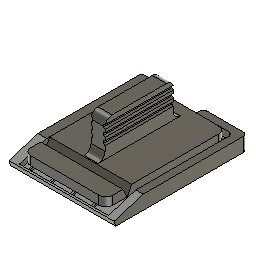
shadowmask_quadrant_cleaver (Autodesk Fusion 360 design; units mm, degrees)
Autodesk Fusion 360 part; units mm, degrees
note: some values were not read from the file. Chosen so that the rebuilt part matches the saved one: a direction; which face or edge a step refers to. Set by a fixed rule: which sketch regions a step uses.
sketch "Sketch1" plane through (0, 0, 0) normal (0, 0, 1) x (1, 0, 0)
  line L0 (39.6677, 30.4381) -> (40.9576, 28.6788)
  line L1 (46.9846, 17.101) -> (47.6858, 15.0353)
  line L2 (10.822, 48.8148) -> (12.941, 48.2963)
  line L3 (35.3553, 35.3553) -> (36.8639, 33.7795)
  line L4 (30.5, 19) -> (26.5, 19)
  line L5 (5.5, 7) -> (5.5, 13)
  line L6 (28.6788, 40.9576) -> (30.4381, 39.6677)
  line L7 (33.7795, 36.8639) -> (35.3553, 35.3553)
  line L8 (4.3578, 49.8097) -> (6.5263, 49.5722)
  line L9 (50, 0) -> (0, 0)
  line L10 (32.1394, 38.3022) -> (33.7795, 36.8639)
  line L11 (2.181, 49.9524) -> (4.3578, 49.8097)
  line L12 (19.1342, 46.194) -> (21.1309, 45.3154)
  line L13 (48.8148, 10.822) -> (49.2404, 8.6824)
  line L14 (12.941, 48.2963) -> (15.0353, 47.6858)
  line L15 (48.2963, 12.941) -> (48.8148, 10.822)
  line L16 (5.5, 13) -> (9.5, 13)
  line L17 (17.101, 46.9846) -> (19.1342, 46.194)
  line L18 (44.3505, 23.0874) -> (45.3154, 21.1309)
  line L19 (49.2404, 8.6824) -> (49.5722, 6.5263)
  line L20 (6.5263, 49.5722) -> (8.6824, 49.2404)
  line L21 (30.4381, 39.6677) -> (32.1394, 38.3022)
  line L22 (0, 0) -> (0, 50)
  line L23 (43.3013, 25) -> (44.3505, 23.0874)
  line L24 (26.5, 19) -> (26.5, 25)
  line L25 (23.0874, 44.3505) -> (25, 43.3013)
  line L26 (42.1696, 26.865) -> (43.3013, 25)
  line L27 (38.3022, 32.1394) -> (39.6677, 30.4381)
  line L28 (49.9524, 2.181) -> (50, 0)
  line L29 (26.5, 25) -> (30.5, 25)
  line L30 (30.5, 25) -> (30.5, 19)
  line L31 (36.8639, 33.7795) -> (38.3022, 32.1394)
  line L32 (21.1309, 45.3154) -> (23.0874, 44.3505)
  line L33 (0, 50) -> (2.181, 49.9524)
  line L34 (46.194, 19.1342) -> (46.9846, 17.101)
  line L35 (40.9576, 28.6788) -> (42.1696, 26.865)
  line L36 (8.6824, 49.2404) -> (10.822, 48.8148)
  line L37 (9.5, 7) -> (5.5, 7)
  line L38 (49.5722, 6.5263) -> (49.8097, 4.3578)
  line L39 (49.8097, 4.3578) -> (49.9524, 2.181)
  line L40 (26.865, 42.1696) -> (28.6788, 40.9576)
  line L41 (47.6858, 15.0353) -> (48.2963, 12.941)
  line L42 (25, 43.3013) -> (26.865, 42.1696)
  line L43 (45.3154, 21.1309) -> (46.194, 19.1342)
  line L44 (15.0353, 47.6858) -> (17.101, 46.9846)
  line L45 (9.5, 13) -> (9.5, 7)
  line L46 (25.0885, 2) -> (24.9115, 2)
  line L47 (17.9115, 4.0885) -> (18.0885, 4.0885)
  line L48 (45.9115, 3.9115) -> (39.0885, 3.9115)
  line L49 (38.9115, 15.9115) -> (32.0885, 15.9115)
  line L50 (45.2548, 15.9115) -> (39.0885, 15.9115)
  line L51 (3.9115, 27.9115) -> (2, 27.9115)
  line L52 (2, 39.9115) -> (3.9115, 39.9115)
  line L53 (10.9115, 16.0885) -> (11.0885, 16.0885)
  line L54 (38.9872, 27.9821) -> (39.0885, 27.9821)
  line L55 (3.9115, 16.0885) -> (3.9115, 27.9115)
  line L56 (2, 4.0885) -> (3.9115, 4.0885)
  line L57 (25.0885, 28.0885) -> (31.9115, 28.0885)
  line L58 (4.0885, 39.9115) -> (10.9115, 39.9115)
  line L59 (26.533, 40.0885) -> (26.533, 39.9115)
  line L60 (24.9115, 16.0885) -> (24.9115, 15.9115)
  line L61 (25.0885, 39.9115) -> (25.0885, 28.0885)
  line L62 (11.0885, 28.0885) -> (17.9115, 28.0885)
  line L63 (45.9115, 2) -> (45.9115, 3.9115)
  line L64 (11.0885, 27.9115) -> (17.9115, 27.9115)
  line L65 (10.9115, 28.0885) -> (10.9115, 39.9115)
  line L66 (17.9115, 39.9115) -> (11.0885, 39.9115)
  line L67 (4.0885, 39.9115) -> (4.0885, 28.0885)
  line L68 (10.9115, 15.9115) -> (11.0885, 15.9115)
  line L69 (31.9115, 16.0885) -> (31.9115, 27.9115)
  line L70 (18.0885, 39.9115) -> (18.0885, 28.0885)
  line L71 (3.9115, 28.0885) -> (3.9115, 39.9115)
  line L72 (3.9115, 16.0885) -> (3.9115, 15.9115)
  line L73 (32.0885, 4.0885) -> (38.9115, 4.0885)
  line L74 (10.9115, 16.0885) -> (10.9115, 27.9115)
  line L75 (2, 3.9115) -> (2, 4.0885)
  line L76 (4.0885, 15.9115) -> (4.0885, 4.0885)
  line L77 (4.0885, 16.0885) -> (3.9115, 16.0885)
  line L78 (38.9872, 27.9115) -> (38.9872, 27.9821)
  line L79 (39.0885, 4.0885) -> (38.9115, 4.0885)
  line L80 (3.9115, 47.833) -> (4.0885, 47.833)
  line L81 (10.9115, 4.0885) -> (11.0885, 4.0885)
  line L82 (4.0885, 28.0885) -> (10.9115, 28.0885)
  line L83 (4.0885, 27.9115) -> (10.9115, 27.9115)
  line L84 (3.9115, 4.0885) -> (4.0885, 4.0885)
  line L85 (18.0885, 40.0885) -> (17.9115, 40.0885)
  line L86 (2, 39.9115) -> (2, 40.0885)
  line L87 (4.0885, 4.0885) -> (10.9115, 4.0885)
  line L88 (11.0885, 39.9115) -> (17.9115, 39.9115)
  line L89 (38.9115, 3.9115) -> (32.0885, 3.9115)
  line L90 (39.0885, 16.0885) -> (38.9115, 16.0885)
  line L91 (17.9115, 16.0885) -> (17.9115, 27.9115)
  line L92 (10.9115, 15.9115) -> (4.0885, 15.9115)
  line L93 (4.0885, 40.0885) -> (10.9115, 40.0885)
  line L94 (31.9115, 15.9115) -> (25.0885, 15.9115)
  line L95 (18.0885, 15.9115) -> (18.0885, 4.0885)
  line L96 (25.0885, 27.9115) -> (25.0885, 16.0885)
  line L97 (11.0885, 4.0885) -> (10.9115, 4.0885)
  line L98 (11.0885, 15.9115) -> (11.0885, 4.0885)
  line L99 (39.0885, 3.9115) -> (39.0885, 4.0885)
  line L100 (4.0885, 15.9115) -> (4.0885, 16.0885)
  line L101 (11.0885, 40.0885) -> (17.9115, 40.0885)
  line L102 (24.9115, 3.9115) -> (18.0885, 3.9115)
  line L103 (11.0885, 40.0885) -> (10.9115, 40.0885)
  line L104 (18.0885, 4.0885) -> (17.9115, 4.0885)
  line L105 (18.0885, 16.0885) -> (24.9115, 16.0885)
  line L106 (24.9115, 39.9115) -> (25.0885, 39.9115)
  line L107 (10.9115, 40.0885) -> (10.9115, 46.7226)
  line L108 (32.0885, 2) -> (31.9115, 2)
  line L109 (31.9115, 4.0885) -> (32.0885, 4.0885)
  line L110 (10.9115, 27.9115) -> (4.0885, 27.9115)
  line L111 (24.9115, 3.9115) -> (18.0885, 3.9115)
  line L112 (18.0885, 15.9115) -> (18.0885, 16.0885)
  line L113 (11.0885, 16.0885) -> (10.9115, 16.0885)
  line L114 (38.9115, 27.9115) -> (32.0885, 27.9115)
  line L115 (31.9115, 16.0885) -> (31.9115, 15.9115)
  line L116 (10.9115, 39.9115) -> (4.0885, 39.9115)
  line L117 (25.0885, 27.9115) -> (25.0885, 28.0885)
  line L118 (31.9115, 28.0885) -> (31.9115, 27.9115)
  line L119 (39.0885, 4.0885) -> (45.9115, 4.0885)
  line L120 (32.0885, 15.9115) -> (32.0885, 16.0885)
  line L121 (3.9115, 4.0885) -> (3.9115, 3.9115)
  line L122 (3.9115, 16.0885) -> (4.0885, 16.0885)
  line L123 (25.0885, 39.9115) -> (25.0885, 40.0885)
  line L124 (18.0885, 28.0885) -> (24.9115, 28.0885)
  line L125 (17.9115, 28.0885) -> (17.9115, 27.9115)
  line L126 (24.9115, 27.9115) -> (18.0885, 27.9115)
  line L127 (38.9115, 27.9821) -> (38.9115, 27.9115)
  line L128 (17.9115, 28.0885) -> (17.9115, 39.9115)
  line L129 (18.0885, 16.0885) -> (17.9115, 16.0885)
  line L130 (32.0885, 28.0885) -> (31.9115, 28.0885)
  line L131 (18.0885, 16.0885) -> (17.9115, 16.0885)
  line L132 (10.9115, 28.0885) -> (10.9115, 27.9115)
  line L133 (38.9115, 16.0885) -> (38.9115, 27.9115)
  line L134 (17.9115, 44.4972) -> (18.0885, 44.4972)
  line L135 (24.9115, 28.0885) -> (24.9115, 27.9115)
  line L136 (24.9115, 15.9115) -> (18.0885, 15.9115)
  line L137 (38.9872, 28.0885) -> (38.9872, 27.9821)
  line L138 (18.0885, 39.9115) -> (18.0885, 40.0885)
  line L139 (39.0885, 15.9115) -> (39.0885, 4.0885)
  line L140 (10.9115, 16.0885) -> (10.9115, 15.9115)
  line L141 (24.9115, 40.9756) -> (25.0885, 40.9756)
  line L142 (4.0885, 4.0885) -> (3.9115, 4.0885)
  line L143 (18.0885, 27.9115) -> (18.0885, 16.0885)
  line L144 (4.0885, 40.0885) -> (3.9115, 40.0885)
  line L145 (32.0885, 4.0885) -> (31.9115, 4.0885)
  line L146 (17.9115, 40.0885) -> (17.9115, 44.4972)
  line L147 (31.9115, 27.9115) -> (25.0885, 27.9115)
  line L148 (25.0885, 27.9115) -> (31.9115, 27.9115)
  line L149 (38.9115, 3.9115) -> (32.0885, 3.9115)
  line L150 (2, 40.0885) -> (3.9115, 40.0885)
  line L151 (18.0885, 4.0885) -> (24.9115, 4.0885)
  line L152 (45.9115, 4.0885) -> (45.9115, 3.9115)
  line L153 (11.0885, 4.0885) -> (17.9115, 4.0885)
  line L154 (17.9115, 16.0885) -> (18.0885, 16.0885)
  line L155 (4.0885, 47.833) -> (4.0885, 40.0885)
  line L156 (4.0885, 3.9115) -> (4.0885, 4.0885)
  line L157 (4.0885, 28.0885) -> (3.9115, 28.0885)
  line L158 (17.9115, 27.9115) -> (11.0885, 27.9115)
  line L159 (10.9115, 39.9115) -> (11.0885, 39.9115)
  line L160 (47.833, 4.0885) -> (47.833, 3.9115)
  line L161 (24.9115, 16.0885) -> (24.9115, 27.9115)
  line L162 (11.0885, 16.0885) -> (10.9115, 16.0885)
  line L163 (17.9115, 15.9115) -> (18.0885, 15.9115)
  line L164 (17.9115, 4.0885) -> (17.9115, 3.9115)
  line L165 (38.9115, 27.9115) -> (32.0885, 27.9115)
  line L166 (18.0885, 3.9115) -> (18.0885, 4.0885)
  line L167 (31.9115, 3.9115) -> (25.0885, 3.9115)
  line L168 (4.0885, 16.0885) -> (10.9115, 16.0885)
  line L169 (3.9115, 15.9115) -> (4.0885, 15.9115)
  line L170 (3.9115, 39.9115) -> (4.0885, 39.9115)
  line L171 (10.9115, 15.9115) -> (4.0885, 15.9115)
  line L172 (25.0885, 15.9115) -> (25.0885, 16.0885)
  line L173 (10.9115, 3.9115) -> (4.0885, 3.9115)
  line L174 (24.9115, 16.0885) -> (25.0885, 16.0885)
  line L175 (18.0885, 28.0885) -> (17.9115, 28.0885)
  line L176 (4.0885, 15.9115) -> (10.9115, 15.9115)
  line L177 (10.9115, 27.9115) -> (11.0885, 27.9115)
  line L178 (25.0885, 40.0885) -> (26.533, 40.0885)
  line L179 (11.0885, 39.9115) -> (11.0885, 40.0885)
  line L180 (47.833, 3.9115) -> (46.0885, 3.9115)
  line L181 (25.0885, 3.9115) -> (25.0885, 4.0885)
  line L182 (11.0885, 46.7226) -> (11.0885, 40.0885)
  line L183 (38.9115, 15.9115) -> (39.0885, 15.9115)
  line L184 (24.9115, 4.0885) -> (24.9115, 3.9115)
  line L185 (25.0885, 16.0885) -> (31.9115, 16.0885)
  line L186 (31.9115, 3.9115) -> (25.0885, 3.9115)
  line L187 (25.0885, 16.0885) -> (24.9115, 16.0885)
  line L188 (10.9115, 4.0885) -> (10.9115, 3.9115)
  line L189 (46.0885, 4.0885) -> (47.833, 4.0885)
  line L190 (4.0885, 16.0885) -> (3.9115, 16.0885)
  line L191 (17.9115, 39.9115) -> (18.0885, 39.9115)
  line L192 (2, 27.9115) -> (3.9115, 27.9115)
  line L193 (11.0885, 28.0885) -> (10.9115, 28.0885)
  line L194 (32.0885, 27.9115) -> (38.9115, 27.9115)
  line L195 (24.9115, 15.9115) -> (25.0885, 15.9115)
  line L196 (2, 28.0885) -> (3.9115, 28.0885)
  line L197 (24.9115, 4.0885) -> (25.0885, 4.0885)
  line L198 (18.0885, 27.9115) -> (18.0885, 28.0885)
  line L199 (32.0885, 16.0885) -> (38.9115, 16.0885)
  line L200 (3.9115, 27.9115) -> (2, 27.9115)
  line L201 (32.0885, 35.7771) -> (32.0885, 28.0885)
  line L202 (38.9115, 16.0885) -> (38.9115, 15.9115)
  line L203 (25.0885, 28.0885) -> (24.9115, 28.0885)
  line L204 (25.0885, 4.0885) -> (24.9115, 4.0885)
  line L205 (2, 16.0885) -> (3.9115, 16.0885)
  line L206 (39.0885, 3.9115) -> (39.0885, 2)
  line L207 (10.9115, 39.9115) -> (4.0885, 39.9115)
  line L208 (25.0885, 4.0885) -> (24.9115, 4.0885)
  line L209 (46.0885, 3.9115) -> (46.0885, 2)
  line L210 (3.9115, 28.0885) -> (3.9115, 27.9115)
  line L211 (24.9115, 4.0885) -> (24.9115, 15.9115)
  line L212 (10.9115, 27.9115) -> (4.0885, 27.9115)
  line L213 (17.9115, 15.9115) -> (11.0885, 15.9115)
  line L214 (32.0885, 27.9115) -> (32.0885, 28.0885)
  line L215 (4.0885, 28.0885) -> (3.9115, 28.0885)
  line L216 (17.9115, 15.9115) -> (11.0885, 15.9115)
  line L217 (10.9115, 46.7226) -> (11.0885, 46.7226)
  line L218 (38.9115, 2) -> (38.9115, 3.9115)
  line L219 (24.9115, 15.9115) -> (18.0885, 15.9115)
  line L220 (38.9115, 27.9115) -> (38.9872, 27.9115)
  line L221 (17.9115, 40.0885) -> (17.9115, 39.9115)
  line L222 (32.0885, 15.9115) -> (32.0885, 4.0885)
  line L223 (11.0885, 39.9115) -> (11.0885, 28.0885)
  line L224 (10.9115, 40.0885) -> (10.9115, 39.9115)
  line L225 (3.9115, 40.0885) -> (3.9115, 47.833)
  line L226 (31.9115, 27.9115) -> (25.0885, 27.9115)
  line L227 (31.9115, 16.0885) -> (32.0885, 16.0885)
  line L228 (38.9115, 3.9115) -> (39.0885, 3.9115)
  line L229 (24.9115, 28.0885) -> (24.9115, 39.9115)
  line L230 (3.9115, 4.0885) -> (3.9115, 15.9115)
  line L231 (24.9115, 27.9115) -> (25.0885, 27.9115)
  line L232 (24.9115, 40.0885) -> (24.9115, 39.9115)
  line L233 (4.0885, 27.9115) -> (4.0885, 16.0885)
  line L234 (46.0885, 4.0885) -> (45.9115, 4.0885)
  line L235 (18.0885, 28.0885) -> (17.9115, 28.0885)
  line L236 (17.9115, 27.9115) -> (11.0885, 27.9115)
  line L237 (24.9115, 2) -> (24.9115, 3.9115)
  line L238 (11.0885, 16.0885) -> (17.9115, 16.0885)
  line L239 (45.9115, 4.0885) -> (45.9115, 13.7113)
  line L240 (32.0885, 4.0885) -> (31.9115, 4.0885)
  line L241 (17.9115, 16.0885) -> (17.9115, 15.9115)
  line L242 (32.0885, 3.9115) -> (32.0885, 2)
  line L243 (32.0885, 16.0885) -> (31.9115, 16.0885)
  line L244 (3.9115, 27.9115) -> (4.0885, 27.9115)
  line L245 (11.0885, 15.9115) -> (17.9115, 15.9115)
  line L246 (39.0885, 2) -> (38.9115, 2)
  line L247 (17.9115, 28.0885) -> (18.0885, 28.0885)
  line L248 (2, 15.9115) -> (3.9115, 15.9115)
  line L249 (2, 15.9115) -> (2, 16.0885)
  line L250 (18.0885, 27.9115) -> (24.9115, 27.9115)
  line L251 (18.0885, 15.9115) -> (24.9115, 15.9115)
  line L252 (2, 27.9115) -> (2, 28.0885)
  line L253 (46.0885, 2) -> (45.9115, 2)
  line L254 (46.0885, 13.7113) -> (46.0885, 4.0885)
  line L255 (25.0885, 40.9756) -> (25.0885, 40.0885)
  line L256 (45.9115, 13.7113) -> (46.0885, 13.7113)
  line L257 (18.0885, 4.0885) -> (17.9115, 4.0885)
  line L258 (17.9115, 4.0885) -> (17.9115, 15.9115)
  line L259 (3.9115, 28.0885) -> (4.0885, 28.0885)
  line L260 (4.0885, 4.0885) -> (3.9115, 4.0885)
  line L261 (25.0885, 3.9115) -> (25.0885, 2)
  line L262 (17.9115, 27.9115) -> (18.0885, 27.9115)
  line L263 (24.9115, 39.9115) -> (18.0885, 39.9115)
  line L264 (18.0885, 44.4972) -> (18.0885, 40.0885)
  line L265 (32.0885, 3.9115) -> (32.0885, 4.0885)
  line L266 (38.9115, 4.0885) -> (38.9115, 3.9115)
  line L267 (17.9115, 3.9115) -> (11.0885, 3.9115)
  line L268 (31.9115, 27.9115) -> (32.0885, 27.9115)
  line L269 (3.9115, 15.9115) -> (2, 15.9115)
  line L270 (26.533, 39.9115) -> (25.0885, 39.9115)
  line L271 (11.0885, 3.9115) -> (11.0885, 4.0885)
  line L272 (32.0885, 28.0885) -> (38.9872, 28.0885)
  line L273 (31.9115, 28.0885) -> (31.9115, 35.7771)
  line L274 (3.9115, 15.9115) -> (2, 15.9115)
  line L275 (3.9115, 39.9115) -> (2, 39.9115)
  line L276 (4.0885, 39.9115) -> (4.0885, 40.0885)
  line L277 (24.9115, 27.9115) -> (18.0885, 27.9115)
  line L278 (25.0885, 15.9115) -> (25.0885, 4.0885)
  line L279 (4.0885, 27.9115) -> (4.0885, 28.0885)
  line L280 (11.0885, 15.9115) -> (11.0885, 16.0885)
  line L281 (39.0885, 27.9821) -> (39.0885, 16.0885)
  line L282 (31.9115, 4.0885) -> (31.9115, 15.9115)
  line L283 (31.9115, 15.9115) -> (32.0885, 15.9115)
  line L284 (24.9115, 40.0885) -> (24.9115, 40.9756)
  line L285 (25.0885, 4.0885) -> (31.9115, 4.0885)
  line L286 (11.0885, 4.0885) -> (10.9115, 4.0885)
  line L287 (45.9115, 3.9115) -> (46.0885, 3.9115)
  line L288 (31.9115, 15.9115) -> (25.0885, 15.9115)
  line L289 (11.0885, 27.9115) -> (11.0885, 16.0885)
  line L290 (39.0885, 15.9115) -> (39.0885, 16.0885)
  line L291 (3.9115, 3.9115) -> (2, 3.9115)
  line L292 (46.0885, 3.9115) -> (46.0885, 4.0885)
  line L293 (38.9872, 27.9821) -> (38.9115, 27.9821)
  line L294 (11.0885, 27.9115) -> (11.0885, 28.0885)
  line L295 (25.0885, 40.0885) -> (24.9115, 40.0885)
  line L296 (31.9115, 4.0885) -> (31.9115, 3.9115)
  line L297 (18.0885, 40.0885) -> (24.9115, 40.0885)
  line L298 (25.0885, 16.0885) -> (24.9115, 16.0885)
  line L299 (3.9115, 39.9115) -> (2, 39.9115)
  line L300 (32.0885, 16.0885) -> (31.9115, 16.0885)
  line L301 (31.9115, 35.7771) -> (32.0885, 35.7771)
  line L302 (39.0885, 16.0885) -> (45.2548, 16.0885)
  line L303 (25.0885, 15.9115) -> (31.9115, 15.9115)
  line L304 (45.2548, 16.0885) -> (45.2548, 15.9115)
  line L305 (11.0885, 28.0885) -> (10.9115, 28.0885)
  line L306 (31.9115, 2) -> (31.9115, 3.9115)
  line L307 (38.9115, 4.0885) -> (38.9115, 15.9115)
  line L308 (3.9115, 40.0885) -> (3.9115, 39.9115)
  line L309 (10.9115, 28.0885) -> (11.0885, 28.0885)
  line L310 (17.9115, 39.9115) -> (11.0885, 39.9115)
  line L311 (10.9115, 4.0885) -> (10.9115, 15.9115)
  line L312 (32.0885, 27.9115) -> (32.0885, 16.0885)
  line L313 (3.9115, 3.9115) -> (2, 3.9115)
  line L314 (3.9115, 2) -> (3.9115, 3.9115)
  line L315 (25.0885, 3.9115) -> (31.9115, 3.9115)
  line L316 (4.0885, 3.9115) -> (10.9115, 3.9115)
  line L317 (2, 3.9115) -> (3.9115, 3.9115)
  line L318 (32.0885, 3.9115) -> (38.9115, 3.9115)
  line L319 (18.0885, 3.9115) -> (24.9115, 3.9115)
  line L320 (31.9115, 3.9115) -> (32.0885, 3.9115)
  line L321 (24.9115, 3.9115) -> (25.0885, 3.9115)
  line L322 (3.9115, 3.9115) -> (4.0885, 3.9115)
  line L323 (17.9115, 3.9115) -> (18.0885, 3.9115)
  line L324 (11.0885, 3.9115) -> (17.9115, 3.9115)
  line L325 (10.9115, 3.9115) -> (11.0885, 3.9115)
  line L326 (30.9081, 25.4081) -> (30.9081, 18.5919)
  line L327 (12.0919, 6.5919) -> (12.0919, 13.4081)
  line L328 (26.0919, 6.5919) -> (26.0919, 13.4081)
  line L329 (11.0885, 3.9115) -> (11.0885, 2)
  line L330 (23.9081, 13.4081) -> (23.9081, 6.5919)
  line L331 (23.9081, 25.4081) -> (23.9081, 18.5919)
  line L332 (10.9115, 3.9115) -> (4.0885, 3.9115)
  line L333 (9.9081, 30.5919) -> (5.0919, 30.5919)
  line L334 (26.0919, 25.4081) -> (30.9081, 25.4081)
  line L335 (16.9081, 13.4081) -> (16.9081, 6.5919)
  line L336 (9.9081, 25.4081) -> (9.9081, 18.5919)
  line L337 (5.0919, 25.4081) -> (9.9081, 25.4081)
  line L338 (5.0919, 18.5919) -> (5.0919, 25.4081)
  line L339 (12.0919, 37.4081) -> (16.9081, 37.4081)
  line L340 (19.0919, 25.4081) -> (23.9081, 25.4081)
  line L341 (16.9081, 30.5919) -> (12.0919, 30.5919)
  line L342 (19.0919, 6.5919) -> (19.0919, 13.4081)
  line L343 (19.0919, 18.5919) -> (19.0919, 25.4081)
  line L344 (4.0885, 2) -> (3.9115, 2)
  line L345 (9.9081, 37.4081) -> (9.9081, 30.5919)
  line L346 (11.0885, 2) -> (10.9115, 2)
  line L347 (26.0919, 13.4081) -> (30.9081, 13.4081)
  line L348 (23.9081, 6.5919) -> (19.0919, 6.5919)
  line L349 (33.0919, 6.5919) -> (33.0919, 13.4081)
  line L350 (37.9081, 13.4081) -> (37.9081, 6.5919)
  line L351 (17.9115, 3.9115) -> (11.0885, 3.9115)
  line L352 (9.9081, 6.5919) -> (5.0919, 6.5919)
  line L353 (10.9115, 2) -> (10.9115, 3.9115)
  line L354 (16.9081, 37.4081) -> (16.9081, 30.5919)
  line L355 (4.0885, 3.9115) -> (4.0885, 2)
  line L356 (12.0919, 13.4081) -> (16.9081, 13.4081)
  line L357 (16.9081, 25.4081) -> (16.9081, 18.5919)
  line L358 (30.9081, 6.5919) -> (26.0919, 6.5919)
  line L359 (5.0919, 6.5919) -> (5.0919, 13.4081)
  line L360 (26.0919, 18.5919) -> (26.0919, 25.4081)
  line L361 (12.0919, 30.5919) -> (12.0919, 37.4081)
  line L362 (23.9081, 37.4081) -> (23.9081, 30.5919)
  line L363 (9.9081, 13.4081) -> (9.9081, 6.5919)
  line L364 (18.0885, 2) -> (17.9115, 2)
  line L365 (19.0919, 30.5919) -> (19.0919, 37.4081)
  line L366 (23.9081, 30.5919) -> (19.0919, 30.5919)
  line L367 (33.0919, 13.4081) -> (37.9081, 13.4081)
  line L368 (19.0919, 37.4081) -> (23.9081, 37.4081)
  line L369 (23.9081, 18.5919) -> (19.0919, 18.5919)
  line L370 (16.9081, 6.5919) -> (12.0919, 6.5919)
  line L371 (17.9115, 2) -> (17.9115, 3.9115)
  line L372 (12.0919, 18.5919) -> (12.0919, 25.4081)
  line L373 (19.0919, 13.4081) -> (23.9081, 13.4081)
  line L374 (16.9081, 18.5919) -> (12.0919, 18.5919)
  line L375 (12.0919, 25.4081) -> (16.9081, 25.4081)
  line L376 (30.9081, 13.4081) -> (30.9081, 6.5919)
  line L377 (18.0885, 3.9115) -> (18.0885, 2)
  line L378 (5.0919, 37.4081) -> (9.9081, 37.4081)
  line L379 (37.9081, 6.5919) -> (33.0919, 6.5919)
  line L380 (30.9081, 18.5919) -> (26.0919, 18.5919)
  line L381 (9.9081, 18.5919) -> (5.0919, 18.5919)
  line L382 (5.0919, 13.4081) -> (9.9081, 13.4081)
  line L383 (5.0919, 30.5919) -> (5.0919, 37.4081)
sketch "Sketch2" plane through (0, 0, 0) normal (0, 0, 1) x (1, 0, 0)
  line L0 (-5, 55) -> (55, 55)
  line L1 (55, 55) -> (55, -19.9471)
  line L2 (55, -19.9471) -> (-5, -19.9471)
  line L3 (-5, -19.9471) -> (-5, 55)
  constraint horizontal L0
  constraint vertical L1
  constraint horizontal L2
  constraint vertical L3
extrude "Extrude1" add sketch "Sketch2" along normal blind 8 makes body 1
sketch "Sketch3" plane through (0, 0, 8) normal (0, 0, 1) x (-1, 0, 0)
  line L0 (5, 19.9471) -> (-55, 19.9471)
  line L1 (-55, 19.9471) -> (-55, -55)
  line L2 (-55, -55) -> (5, -55)
  line L3 (5, -55) -> (5, 19.9471)
  line L4 (5, -55) -> (0, -55)
  line L5 (0, -55) -> (0, 19.9471)
  line L6 (0, 19.9471) -> (5, 19.9471)
  line L7 (5, 19.9471) -> (5, -55)
  line L8 (-55, 19.9471) -> (-50.82, 19.9471)
  line L9 (-50.82, 19.9471) -> (-50.82, -55)
  line L10 (-50.82, -55) -> (-55, -55)
  line L11 (-55, -55) -> (-55, 19.9471)
  line L12 (0, -55) -> (-50.82, -55)
  line L13 (-50.82, -55) -> (-50.82, -51)
  line L14 (-50.82, -51) -> (0, -51)
  line L15 (0, -51) -> (0, -55)
  constraint horizontal L4
  constraint vertical L5
  constraint horizontal L6
  constraint vertical L7
  constraint coincident L0 L5.end
  constraint coincident L2.end L3.start
  constraint horizontal L8
  constraint vertical L9
  constraint horizontal L10
  constraint vertical L11
  constraint coincident L2 L9.end
  constraint coincident L0.end L1.start
  constraint horizontal L12
  constraint vertical L13
  constraint horizontal L14
  constraint vertical L15
  constraint coincident L9 L13.end
  constraint coincident origin L5
extrude "Extrude2" cut sketch "Sketch3" against normal blind 3 contours L0 L5 L9 L14 bodies 1
sketch "Sketch4" plane through (0, 0, 8) normal (0, 0, 1) x (-1, 0, 0)
  line L0 (-50.82, -51) -> (-50.82, 19.9471)
  line L1 (-50.82, 19.9471) -> (-55, 19.9471)
  line L2 (-55, 19.9471) -> (-55, -55)
  line L3 (-55, -55) -> (5, -55)
  line L4 (5, -55) -> (5, 19.9471)
  line L5 (5, 19.9471) -> (0, 19.9471)
  line L6 (0, 19.9471) -> (0, -51)
  line L7 (0, -51) -> (-50.82, -51)
  line L8 (0, -55) -> (-30, -55)
  line L9 (-30, -55) -> (-30, -43)
  line L10 (-30, -43) -> (0, -43)
  line L11 (0, -43) -> (0, -55)
  dimension "d7" = 30
  constraint horizontal L8
  constraint vertical L9
  constraint horizontal L10
  constraint vertical L11
  constraint coincident L3 L8.start
  constraint coincident L6 L10.end
  measures "d7" distance of L9 L11
extrude "Extrude3" cut sketch "Sketch4" against normal blind 10 contours L6 L7 L9 L10 L11 | L3 L7 L8 L9 L11 bodies 1
sketch "Sketch5" plane through (0, 0, 5) normal (0, 0, 1) x (-1, 0, 0)
  line L0 (-30, -51) -> (-30, -43)
  line L1 (-30, -43) -> (0, -43)
  line L2 (0, -43) -> (0, 19.9471)
  line L3 (0, 19.9471) -> (-50.82, 19.9471)
  line L4 (-50.82, 19.9471) -> (-50.82, -51)
  line L5 (-50.82, -51) -> (-30, -51)
  line L6 (-3.4885, -43) -> (-4.4885, -43)
  line L7 (-4.4885, -43) -> (-4.4885, 19.9471)
  line L8 (-4.4885, 19.9471) -> (-3.4885, 19.9471)
  line L9 (-3.4885, 19.9471) -> (-3.4885, -43)
  line L10 (-4.0885, -3.9115) -> (-4.0885, -2)
  line L11 (-16.4885, -43) -> (-16.4885, 19.9471)
  line L12 (-16.0885, -3.9115) -> (-16.0885, -2)
  line L13 (-15.4885, -43) -> (-16.4885, -43)
  line L14 (-15.4885, 19.9471) -> (-15.4885, -43)
  line L15 (-16.4885, 19.9471) -> (-15.4885, 19.9471)
  line L16 (-28.4885, -43) -> (-28.4885, 19.9471)
  line L17 (-28.0885, -3.9115) -> (-28.0885, -2)
  line L18 (-27.4885, -43) -> (-28.4885, -43)
  line L19 (-27.4885, 19.9471) -> (-27.4885, -43)
  line L20 (-28.4885, 19.9471) -> (-27.4885, 19.9471)
  line L21 (-40.4885, -43) -> (-40.4885, 19.9471)
  line L22 (-40.0885, -3.9115) -> (-40.0885, -2)
  line L23 (-39.4885, -43) -> (-40.4885, -43)
  line L24 (-39.4885, 19.9471) -> (-39.4885, -43)
  line L25 (-40.4885, 19.9471) -> (-39.4885, 19.9471)
  dimension "d8" = 1
  dimension "d9" = 0.4
  dimension "d12" = -12
  dimension "d13" = 0
  constraint horizontal L6
  constraint vertical L7
  constraint horizontal L8
  constraint vertical L9
  constraint coincident L3 L7.end
  constraint coincident L1 L6.start
  measures "d8" distance of L7 L9
  measures "d9" distance of L7 L10
extrude "Extrude4" cut sketch "Sketch5" against normal blind 1 contours L0 L1 L3 L4 L5 L16 L21 L23 L24 | L1 L3 L11 L19 | L1 L3 L7 L14 | L1 L2 L3 L9 bodies 1
sketch "Sketch6" plane through (55, 0, 0) normal (1, 0, 0) x (0, 1, 0)
  line L0 (-19.9471, 0) -> (55, 0)
  line L1 (55, 0) -> (55, 8)
  line L2 (55, 8) -> (-19.9471, 8)
  line L3 (-19.9471, 8) -> (-19.9471, 0)
  line L4 (-19.9471, 0) -> (5.8405, 8)
  dimension "d27" = 27
  constraint coincident L0.start L3.end
  constraint coincident L2 L4.end
  measures "d27" distance of L0.start L4.end
extrude "Extrude5" cut sketch "Sketch6" against normal blind 100 contours L2 L3 L4 bodies 1
fillet "Fillet2" radius 2 2 edges at (-5, 55, 4) (55, 55, 4) on bodies 1
fillet "Fillet2" radius 2 4 edges at (0, 55, 4) (30, 55, 4) (0, 43, 2) (30, 43, 2) on bodies 1
fillet "Fillet2" radius 2 1 edges at (50.82, 51, 6) on bodies 1
chamfer "Chamfer1" distance 1 angle 45 5 edges at (39.9885, 43, 5) (27.7443, 43, 5) (28.2461, 43.0152, 5) (15.9885, 43, 5) (3.9885, 43, 5) on bodies 1
sketch "Sketch7" plane through (0, -1.7512, 5.6449) normal (0, -0.296296, 0.955096) x (1, 0, 0)
  line L0 (50.82, 7.9486) -> (50.82, -5.5514)
  line L1 (50.82, -5.5514) -> (40.4885, -5.5514)
  line L2 (40.4885, -5.5514) -> (40.4885, -2.1764)
  line L3 (40.4885, -2.1764) -> (39.4885, -2.1764)
  line L4 (39.4885, -2.1764) -> (39.4885, -5.5514)
  line L5 (39.4885, -5.5514) -> (28.4885, -5.5514)
  line L6 (28.4885, -5.5514) -> (28.4885, -2.1764)
  line L7 (28.4885, -2.1764) -> (27.4885, -2.1764)
  line L8 (27.4885, -2.1764) -> (27.4885, -5.5514)
  line L9 (27.4885, -5.5514) -> (16.4885, -5.5514)
  line L10 (16.4885, -5.5514) -> (16.4885, -2.1764)
  line L11 (16.4885, -2.1764) -> (15.4885, -2.1764)
  line L12 (15.4885, -2.1764) -> (15.4885, -5.5514)
  line L13 (15.4885, -5.5514) -> (4.4885, -5.5514)
  line L14 (4.4885, -5.5514) -> (4.4885, -2.1764)
  line L15 (4.4885, -2.1764) -> (3.4885, -2.1764)
  line L16 (3.4885, -2.1764) -> (3.4885, -5.5514)
  line L17 (3.4885, -5.5514) -> (0, -5.5514)
  line L18 (0, -5.5514) -> (0, 7.9486)
  line L19 (0, 7.9486) -> (-5, 7.9486)
  line L20 (-5, 7.9486) -> (-5, -19.0514)
  line L21 (-5, -19.0514) -> (55, -19.0514)
  line L22 (55, -19.0514) -> (55, 7.9486)
  line L23 (55, 7.9486) -> (50.82, 7.9486)
  line L24 (3.4885, -2.1764) -> (4.4885, -2.1764)
  line L25 (4.4885, -2.1764) -> (4.4885, -19.0514)
  line L26 (4.4885, -19.0514) -> (3.4885, -19.0514)
  line L27 (3.4885, -19.0514) -> (3.4885, -2.1764)
  line L28 (15.4885, -19.0514) -> (15.4885, -2.1764)
  line L29 (16.4885, -2.1764) -> (16.4885, -19.0514)
  line L30 (15.4885, -2.1764) -> (16.4885, -2.1764)
  line L31 (16.4885, -19.0514) -> (15.4885, -19.0514)
  line L32 (27.4885, -19.0514) -> (27.4885, -2.1764)
  line L33 (28.4885, -2.1764) -> (28.4885, -19.0514)
  line L34 (27.4885, -2.1764) -> (28.4885, -2.1764)
  line L35 (28.4885, -19.0514) -> (27.4885, -19.0514)
  line L36 (39.4885, -19.0514) -> (39.4885, -2.1764)
  line L37 (40.4885, -2.1764) -> (40.4885, -19.0514)
  line L38 (39.4885, -2.1764) -> (40.4885, -2.1764)
  line L39 (40.4885, -19.0514) -> (39.4885, -19.0514)
  line L40 (50.82, 7.9486) -> (55, 7.9486)
  line L41 (55, 7.9486) -> (55, -19.0514)
  line L42 (55, -19.0514) -> (50.82, -19.0514)
  line L43 (50.82, -19.0514) -> (50.82, 7.9486)
  line L44 (0, 7.9486) -> (-5, 7.9486)
  line L45 (-5, 7.9486) -> (-5, -19.0514)
  line L46 (-5, -19.0514) -> (0, -19.0514)
  line L47 (0, -19.0514) -> (0, 7.9486)
  dimension "d30" = 12
  dimension "d31" = 0
  constraint horizontal L24
  constraint vertical L25
  constraint horizontal L26
  constraint vertical L27
  constraint coincident L21 L25.end
  constraint coincident L15.end L16.start
  constraint horizontal L40
  constraint vertical L41
  constraint horizontal L42
  constraint vertical L43
  constraint coincident L21.end L22.start
  constraint coincident L0.start L23.end
  constraint horizontal L44
  constraint vertical L45
  constraint horizontal L46
  constraint vertical L47
  constraint coincident L20.end L21.start
  constraint coincident L18.end L19.start
  constraint coincident L10.end L29
extrude "Extrude6" add sketch "Sketch7" along normal blind 1 contours L0 L21 L22 L23 L40 L41 L42 L43 | L2 L3 L4 L21 L36 L37 L38 L39 | L6 L7 L8 L21 L32 L33 L34 L35 | L10 L11 L12 L21 L28 L29 L30 L31 | L14 L15 L16 L21 L24 L25 L26 L27 bodies 1
sketch "Sketch8" plane through (51.4885, 0, 0) normal (1, 0, 0) x (0, 1, 0)
  line L0 (-3.8298, 5) -> (-4.1261, 5.9551)
  line L1 (-4.1261, 5.9551) -> (-20.2434, 0.9551)
  line L2 (-20.2434, 0.9551) -> (-19.9471, 0)
  line L3 (-19.9471, 0) -> (-3.8298, 5)
  line L4 (-3.8298, 5) -> (-7.2048, 5)
  constraint coincident L0.start L3.end
  constraint coincident L1 L4.end
extrude "Extrude7" cut sketch "Sketch8" against normal blind 100 contours L0 L1 L4 bodies 1
sketch "Sketch9" plane through (0, -1.7512, 5.6449) normal (0, -0.296296, 0.955096) x (1, 0, 0)
  line L0 (40.4885, -19.0514) -> (50.82, -19.0514)
  line L1 (50.82, -19.0514) -> (50.82, -5.5514)
  line L2 (-5, 7.9486) -> (0, 7.9486)
  line L3 (0, 7.9486) -> (0, -18.0514)
  line L4 (0, -18.0514) -> (-5, -18.0514)
  line L5 (-5, -18.0514) -> (-5, 7.9486)
  line L6 (50.82, 7.9486) -> (55, 7.9486)
  line L7 (55, 7.9486) -> (55, -19.0514)
  line L8 (55, -19.0514) -> (50.82, -19.0514)
  line L9 (50.82, -19.0514) -> (50.82, 7.9486)
  line L10 (55, -19.0514) -> (-5, -19.0514)
  line L11 (-5, -19.0514) -> (-5, -18.0514)
  line L12 (-5, -18.0514) -> (55, -18.0514)
  line L13 (55, -18.0514) -> (55, -19.0514)
  line L14 (-5, 7.9486) -> (0, 7.9486)
  line L15 (50.82, -5.5514) -> (40.4885, -5.5514)
  line L16 (40.4885, -5.5514) -> (40.4885, -19.0514)
  dimension "d40" = 1
  constraint horizontal L2
  constraint vertical L3
  constraint horizontal L4
  constraint vertical L5
  constraint horizontal L6
  constraint vertical L7
  constraint horizontal L8
  constraint vertical L9
  constraint coincident L0.end L7.end
  constraint coincident L0.end L6.start
  constraint horizontal L10
  constraint vertical L11
  constraint horizontal L12
  constraint vertical L13
  constraint coincident L5 L4.end
  constraint coincident L2.end L14
  constraint coincident L3.end L12
  measures "d40" distance of L10 L12
extrude "Extrude8" add sketch "Sketch9" along normal blind 3 contours L0 L1 L9 L10 L12 L16 | L4 L10 L11 L12 L16 | L1 L7 L8 L9 L10 L12 L13 | L1 L6 L7 L9 L12 | L2 L3 L4 L5 L12 L14 bodies 1
sketch "Sketch10" plane through (55, 0, 0) normal (1, 0, 0) x (0, 1, 0)
  line L0 (53, 0) -> (53, 8)
  line L1 (53, 8) -> (5.8405, 8)
  line L2 (5.8405, 8) -> (4.9516, 10.8653)
  line L3 (4.9516, 10.8653) -> (-20.836, 2.8653)
  line L4 (-20.836, 2.8653) -> (-19.9471, 0)
  line L5 (-19.9471, 0) -> (53, 0)
  line L6 (5.8405, 8) -> (-8.0281, 8)
  line L7 (-8.0281, 8) -> (-8.0281, 11.5741)
  line L8 (-8.0281, 11.5741) -> (5.8405, 11.5741)
  line L9 (5.8405, 11.5741) -> (5.8405, 8)
  constraint horizontal L6
  constraint vertical L7
  constraint horizontal L8
  constraint vertical L9
  constraint coincident L1.end L2.start
extrude "Extrude9" cut sketch "Sketch10" against normal blind 1000 contours L2 L3 L6 bodies 1
copy_body "Body->Comp1" bodies 1 removing the originals makes body 2 in component "Component"
sketch "Sketch1 (2)" plane through (0, 0, 5) normal (0, 0, 1) x (-1, 0, 0) in component "Component'"
  line L0 (-3.4885, 7.2048) -> (-4.4885, 7.2048)
  line L1 (-48.82, -49) -> (-2, -49)
  line L2 (-2, -49) -> (-2, 19.3809)
  line L3 (-2, 19.3809) -> (-48.82, 19.3809)
  line L4 (-48.82, 19.3809) -> (-48.82, -49)
  line L5 (0, 0) -> (0, -50)
  line L6 (-50.82, 4.2845) -> (-50.82, -49)
  line L7 (-30, -51) -> (-48.82, -51)
  line L8 (-50.82, 19.8809) -> (0, 19.8809)
  line L9 (-40.4885, 7.2048) -> (-40.4885, -42)
  line L10 (-39.4885, -42) -> (-39.4885, 7.2048)
  line L11 (-4.4885, -42) -> (-3.4885, -42)
  line L12 (-3.4885, -42) -> (-3.4885, 7.2048)
  line L13 (-4.4885, 7.2048) -> (-4.4885, -42)
  line L14 (-40.4885, -42) -> (-39.4885, -42)
  line L15 (-39.4885, 7.2048) -> (-40.4885, 7.2048)
  line L16 (-16.4885, -42) -> (-15.4885, -42)
  line L17 (-15.4885, -42) -> (-15.4885, 7.2048)
  line L18 (-15.4885, 7.2048) -> (-16.4885, 7.2048)
  line L19 (-16.4885, 7.2048) -> (-16.4885, -42)
  dimension "d41" = 2
  dimension "d42" = 2
  dimension "d43" = 2
  dimension "d44" = 0.5
  constraint horizontal L1
  constraint vertical L2
  constraint horizontal L3
  constraint vertical L4
  measures "d41" distance of L2 L5
  measures "d42" distance of L4 L6
  measures "d43" distance of L1 L7
  measures "d44" distance of L3 L8
extrude "Extrude1'" add sketch "Sketch1 (2)" along normal blind 5 separate body contours L0 L11 L12 L13 | L1 L2 L3 L4 | L9 L10 L14 L15 | L16 L17 L18 L19 makes body 3 in component "Component'"
sketch "Sketch2 (2)" plane through (48.82, 0, 0) normal (1, 0, 0) x (0, 1, 0) in component "Component'"
  line L0 (-19.3809, 5) -> (49, 5)
  line L1 (49, 5) -> (49, 10)
  line L2 (49, 10) -> (-19.3809, 10)
  line L3 (-19.3809, 10) -> (-19.3809, 5)
  line L4 (-7.4578, 5.4) -> (-9.6578, 10)
  line L5 (-7.4578, 5.4) -> (-6.8578, 5.4)
  line L6 (-6.8578, 5.4) -> (-4.6578, 10)
  dimension "d47" = 5
  dimension "d48" = 0.6
  dimension "d49" = 0.4
  dimension "d50" = 2.2
  constraint coincident L2 L4.end
  constraint parallel L0 L5
  constraint coincident L2 L6.end
  measures "d47" distance of L4.end L6.end
  measures "d48" distance of L4.start L5.end
  measures "d49" distance of L0 L5
  measures "d50" horizontal distance of L5.end L6.end
extrude "Extrude2'" cut sketch "Sketch2 (2)" against normal blind 100 contours L2 L4 L5 L6 bodies 3 in component "Component'"
sketch "Sketch3 (2)" plane through (0, 0, 10) normal (0, 0, 1) x (-1, 0, 0) in component "Component'"
  line L0 (-2, 4.6578) -> (-48.82, 4.6578)
  line L1 (-48.82, 4.6578) -> (-48.82, -49)
  line L2 (-48.82, -49) -> (-2, -49)
  line L3 (-2, -49) -> (-2, 4.6578)
  line L4 (-21, 0) -> (-29, 0)
  line L5 (-29, 0) -> (-29, -39)
  line L6 (-29, -39) -> (-21, -39)
  line L7 (-21, -39) -> (-21, 0)
  constraint horizontal L4
  constraint vertical L5
  constraint horizontal L6
  constraint vertical L7
extrude "Extrude3'" add sketch "Sketch3 (2)" along normal blind 20 contours L4 L5 L6 L7 bodies 3 in component "Component'"
fillet "Fillet1" radius 4 8 edges at (2, 49, 7.5) (48.82, 49, 7.5) (2, -19.3809, 7.5) (48.82, -19.3809, 7.5) (25, 0, 30) (25, 39, 30) (25, 39, 10) (25, 0, 10) on bodies 3 in component "Component'"
sketch "Sketch4 (2)" plane through (0, 0, 0) normal (0, -1, 0) x (1, 0, 0) in component "Component'"
  line L0 (21, 14) -> (29, 14)
  line L1 (29, 14) -> (29, 26)
  line L2 (29, 26) -> (21, 26)
  line L3 (21, 26) -> (21, 14)
  line L4 (25, 30) -> (25, 14)
  line L5 (22, 26.5774) -> (21, 27.1547)
  line L6 (21, 27.1547) -> (20, 26.5773)
  line L7 (20, 26.5773) -> (20, 25.4226)
  line L8 (20, 25.4226) -> (21, 24.8453)
  line L9 (21, 24.8453) -> (22, 25.4227)
  line L10 (22, 25.4227) -> (22, 26.5774)
  line L11 (22, 22.5774) -> (21, 23.1547)
  line L12 (21, 23.1547) -> (20, 22.5774)
  line L13 (20, 22.5774) -> (20, 21.4227)
  line L14 (20, 21.4227) -> (21, 20.8453)
  line L15 (21, 20.8453) -> (22, 21.4227)
  line L16 (22, 21.4227) -> (22, 22.5774)
  line L17 (22, 18.5774) -> (21, 19.1547)
  line L18 (21, 19.1547) -> (20, 18.5774)
  line L19 (20, 18.5774) -> (20, 17.4226)
  line L20 (20, 17.4226) -> (21, 16.8453)
  line L21 (21, 16.8453) -> (22, 17.4226)
  line L22 (22, 17.4226) -> (22, 18.5774)
  line L23 (30, 22.5774) -> (30, 21.4227)
  line L24 (30, 21.4227) -> (29, 20.8453)
  line L25 (30, 18.5774) -> (30, 17.4226)
  line L26 (28, 26.5774) -> (29, 27.1547)
  line L27 (28, 17.4226) -> (28, 18.5774)
  line L28 (29, 23.1547) -> (30, 22.5774)
  line L29 (28, 25.4227) -> (28, 26.5774)
  line L30 (30, 17.4226) -> (29, 16.8453)
  line L31 (29, 19.1547) -> (30, 18.5774)
  line L32 (29, 24.8453) -> (28, 25.4227)
  line L33 (28, 21.4227) -> (28, 22.5774)
  line L34 (28, 18.5774) -> (29, 19.1547)
  line L35 (29, 16.8453) -> (28, 17.4226)
  line L36 (29, 20.8453) -> (28, 21.4227)
  line L37 (29, 27.1547) -> (30, 26.5773)
  line L38 (28, 22.5774) -> (29, 23.1547)
  line L39 (30, 26.5773) -> (30, 25.4226)
  line L40 (30, 25.4226) -> (29, 24.8453)
  point P0 (21, 26)
  point P1 (21, 22)
  point P2 (21, 18)
  point P3 (29, 26)
  point P4 (29, 26)
  point P5 (29, 22)
  point P6 (29, 18)
  constraint midpoint L0 L4.end
  constraint perpendicular L0 L4
  constraint coincident P0 L2.end
  constraint coincident L3 P1
  constraint coincident L3 P2
  constraint symmetric P0 L4 P3
  constraint symmetric L4 L5.start L26.start
  constraint symmetric L4 L5.end L26.end
  constraint symmetric L4 L6.end L37.end
  constraint symmetric L4 L7.end L39.end
  constraint symmetric L4 L8.end L32.start
  constraint symmetric L4 L9.end L29.start
  constraint symmetric L4 P0 P4
  constraint symmetric L4 L11.start L33.end
  constraint symmetric L4 L11.end L28.start
  constraint symmetric L4 L12.end L23.start
  constraint symmetric L4 L13.end L23.end
  constraint symmetric L4 L14.end L24.end
  constraint symmetric L4 L15.end L33.start
  constraint symmetric L4 P1 P5
  constraint symmetric L4 L17.start L27.end
  constraint symmetric L4 L17.end L31.start
  constraint symmetric L4 L18.end L25.start
  constraint symmetric L4 L19.end L25.end
  constraint symmetric L4 L20.end L30.end
  constraint symmetric L4 L21.end L27.start
  constraint symmetric L4 P2 P6
extrude "Extrude4'" cut sketch "Sketch4 (2)" against normal blind 50 contours L3 L17 L21 L22 | L1 L27 L34 L35 | L1 L2 L26 L29 L37 L39 L40 | L1 L2 L29 L32 | L2 L3 L9 L10 | L2 L3 L5 L6 L7 L8 L10 | L3 L11 L15 L16 | L1 L33 L36 L38 bodies 3 in component "Component'"
component "Component" placed x (1, 0, 0) y (0, 1, 0) z (0, 0, 1) at (0, 0, 0)
component "Component'" placed x (1, 0, 0) y (0, 1, 0) z (0, 0, 1) at (0, 0, 0)
